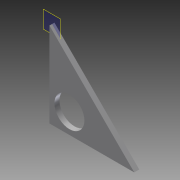
# Autodesk Inventor part: GE-13018-05
Saved by Autodesk Inventor 2013 (Build 170138000, 138)
## iProperties
Created: 2013-01-05
Part Number: GE-13018-05
Material: Steel
Document SubType Name: Modeling
Designer: Phillip
Density: 1 g/cm^3
Author: Phillip
Autodesk Inventor part; units mm, degrees
ref_plane "YZ Plane" through (0, 0, 0) normal (1, 0, 0) x (0, 1, 0)
ref_plane "XZ Plane" through (0, 0, 0) normal (0, 1, 0) x (-1, 0, 0)
ref_plane "XY Plane" through (0, 0, 0) normal (0, 0, 1) x (1, 0, 0)
sketch "Sketch1" plane through (0, 0, 0) normal (0, 0, 1) x (1, 0, 0)
  line L0 (0, 0) -> (107.696, 0)
  line L1 (107.696, 0) -> (0, 107.696)
  line L2 (0, 107.696) -> (0, 0)
  point P0 (25.4, 25.4)
  dimension "d0" = 107.696
  dimension "d1" = 25.4
  dimension "d2" = 25.4
  constraints: 6 end point, 2 perpendicular, 1 horizontal
  measures "d0" distance of L0.start L0.end
  measures "d1" distance from line of point (25.4, 25.4) L0
  measures "d2" distance from line of point (25.4, 25.4) L2
extrude "Extrusion1" add sketch "Sketch1" against normal blind 6.35
hole "Hole1" at (25.4, 25.4, 0) direction (0, 0, -1) diameter 38.1 end through all
ref_plane "Work Plane1" through (0, 107.696, -3.175) normal (0, 0, -1) x (-1, 0, 0)
body "Solid1"
